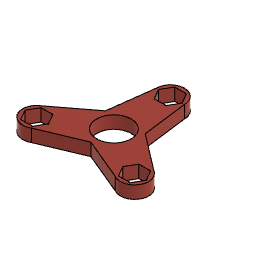
fidget dfab v1 (Autodesk Fusion 360 design; units mm, degrees)
Autodesk Fusion 360 part; units mm, degrees
note: some values were not read from the file. Set by a fixed rule: which sketch regions a step uses.
sketch "Sketch1" plane through (0, 0, 0) normal (0, 0, 1) x (1, 0, 0)
  circle A0 centre (0, 0) radius 4
  circle A1 centre (0, 0) radius 11
  circle A2 centre (0, 0) radius 13.5
  circle A3 centre (0, 36) radius 9
  line L0 (0, 0) -> (0, 45)
  line L1 (-3.7528, 42.5) -> (-7.5056, 36)
  line L2 (-7.5056, 36) -> (-3.7528, 29.5)
  line L3 (-3.7528, 29.5) -> (3.7528, 29.5)
  line L4 (3.7528, 29.5) -> (7.5056, 36)
  line L5 (7.5056, 36) -> (3.7528, 42.5)
  line L6 (3.7528, 42.5) -> (-3.7528, 42.5)
  line L7 (9, 36) -> (13.3906, 1.7148)
  line L8 (-9, 36) -> (-13.3906, 1.7148)
  line L9 (-26.6769, -25.7942) -> (5.2102, -12.4541)
  circle A4 centre (-31.1769, -18) radius 9
  line L10 (-27.4241, -24.5) -> (-23.6714, -18)
  line L11 (-34.9297, -24.5) -> (-27.4241, -24.5)
  line L12 (-38.6825, -18) -> (-34.9297, -24.5)
  line L13 (-27.4241, -11.5) -> (-34.9297, -11.5)
  line L14 (-23.6714, -18) -> (-27.4241, -11.5)
  line L15 (-34.9297, -11.5) -> (-38.6825, -18)
  line L16 (-35.6769, -10.2058) -> (-8.1804, 10.7392)
  line L17 (35.6769, -10.2058) -> (8.1804, 10.7392)
  circle A5 centre (31.1769, -18) radius 9
  line L18 (34.9297, -11.5) -> (27.4241, -11.5)
  line L19 (38.6825, -18) -> (34.9297, -11.5)
  line L20 (34.9297, -24.5) -> (38.6825, -18)
  line L21 (23.6714, -18) -> (27.4241, -24.5)
  line L22 (27.4241, -11.5) -> (23.6714, -18)
  line L23 (27.4241, -24.5) -> (34.9297, -24.5)
  line L24 (26.6769, -25.7942) -> (-5.2102, -12.4541)
  point P0 (0, 36)
  point P1 (0, 36)
  point P2 (0, 36)
  point P3 (0, 36)
  point P4 (0, 36)
  dimension "d1" = 8
  dimension "d2" = 22
  dimension "d3" = 27
  dimension "d10" = 18
  dimension "d12" = 6.5
  dimension "d14" = 360
  constraint coincident A0.centre A1.centre
  constraint concentric A0 A1
  constraint concentric A1 A2
  constraint coincident P3 P2
  constraint coincident P4 P3
  constraint coincident A3 L0.end
  constraint vertical L0
  constraint coincident A3 L7.start
  constraint coincident A2 L7.end
  constraint tangent A2 L7
  constraint coincident A3 L8.start
  constraint coincident A2 L8.end
  constraint tangent A2 L8
  measures "d1" diameter of A0
  measures "d2" diameter of A1
  measures "d3" diameter of A2
  measures "d10" diameter of A3
  measures "d12" distance of P4 L6
extrude "Extrude1" add sketch "Sketch1" along normal blind 8 contours A2 | A2 L7 L9 L17 A5 L24 | A2 L7 L17 | A2 L9 L24 | A2 A3 L0 L7 L17 | A2 L8 L9 A4 L16 L24 | A2 A3 L0 L8 L16 | A3 L0 L3 L4 L5 L6 | A5 | A2 L8 L16 | A4 | A3 L0 L1 L2 L3 L6
